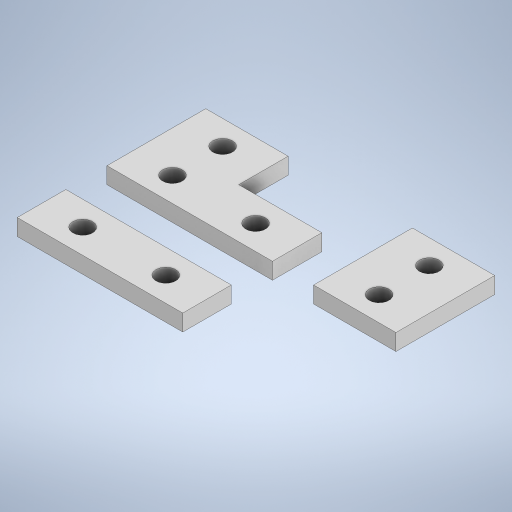
# Autodesk Inventor part: LatchBankGussetSet
Saved by Autodesk Inventor 2024 (Build 280153000, 153)
## iProperties
Created: 2023-11-04
Part Number: LatchBankGussetSet
Material: Generic
Document SubType Name: Modeling
Designer: gcter
Density: 1 g/cm^3
Appearance: Default
Author: gcter
Autodesk Inventor part; units mm, degrees
ref_plane "YZ Plane" through (0, 0, 0) normal (1, 0, 0) x (0, 1, 0)
ref_plane "XZ Plane" through (0, 0, 0) normal (0, 1, 0) x (-1, 0, 0)
ref_plane "XY Plane" through (0, 0, 0) normal (0, 0, 1) x (1, 0, 0)
sketch "Sketch1" plane through (0, 0, 0) normal (0, 1, 0) x (-1, 0, 0)
  line L0 (0, 0) -> (-25.527, 0)
  line L1 (-25.527, 0) -> (-25.527, -7.493)
  line L2 (-25.527, -7.493) -> (0, -7.493)
  line L3 (0, -7.493) -> (0, 0)
  circle A0 centre (-6.35, -3.7465) radius 1.524
  circle A1 centre (-19.177, -3.7465) radius 1.524
  line L4 (-12.7, -21.463) -> (-25.527, -21.463)
  line L5 (-25.527, -21.463) -> (-25.527, -13.843)
  line L6 (-25.527, -13.843) -> (0, -13.843)
  line L7 (0, -13.843) -> (0, -21.463)
  line L8 (0, -29.083) -> (-12.7, -29.083)
  line L9 (-12.7, -29.083) -> (-12.7, -21.463)
  line L10 (0, -21.463) -> (0, -29.083)
  circle A2 centre (-6.35, -17.5895) radius 1.524
  circle A3 centre (-19.177, -17.5895) radius 1.524
  circle A4 centre (-6.35, -25.3365) radius 1.524
  line L11 (-31.877, -13.843) -> (-44.577, -13.843)
  line L12 (-44.577, -13.843) -> (-44.577, -29.083)
  line L13 (-44.577, -29.083) -> (-31.877, -29.083)
  line L14 (-31.877, -29.083) -> (-31.877, -13.843)
  circle A5 centre (-38.227, -17.5895) radius 1.524
  circle A6 centre (-38.227, -25.3365) radius 1.524
  point P0 (-25.527, -17.653)
  dimension "d1" = 7.493
  dimension "d2" = 25.527
  dimension "d3" = 3.048
  dimension "d4" = 3.7465
  dimension "d5" = 6.35
  dimension "d6" = 6.35
  dimension "d8" = 3.048
  dimension "d9" = 6.35
  dimension "d10" = 7.62
  dimension "d11" = 7.62
  dimension "d12" = 12.7
  dimension "d13" = 3.048
  dimension "d14" = 6.35
  dimension "d15" = 3.7465
  dimension "d16" = 3.048
  dimension "d17" = 6.35
  dimension "d18" = 3.048
  dimension "d19" = 3.7465
  dimension "d20" = 12.7
  dimension "d21" = 6.35
  dimension "d22" = 3.048
  dimension "d23" = 6.35
  dimension "d24" = 3.7465
  dimension "d25" = 3.048
  dimension "d26" = 3.7465
  constraints: 30 end point, 7 centre point, 7 parallel, 5 collinear, 4 horizontal, 4 perpendicular, 2 horizontal alignment, 2 vertical alignment, 1 midpoint
  measures "d1" distance between parallel lines of L0 L2
  measures "d2" distance between parallel lines of L1 L3
  measures "d3" diameter of A0
  measures "d4" distance from line of L0 A0.centre
  measures "d5" distance from line of L3 A0.centre
  measures "d6" distance from line of A1.centre L1
  measures "d8" diameter of A1
  measures "d9" distance between parallel lines of L2 L6
  measures "d10" distance between parallel lines of L6 L4
  measures "d11" distance between parallel lines of L4 L8
  measures "d12" distance between parallel lines of L9 L10
  measures "d13" diameter of A2
  measures "d14" distance from line of L7 A2.centre
  measures "d15" distance from line of L6 A2.centre
  measures "d16" diameter of A3
  measures "d17" horizontal distance of point (-25.527, -17.653) A3.centre
  measures "d18" diameter of A4
  measures "d19" distance from line of L8 A4.centre
  measures "d20" distance between parallel lines of L12 L14
  measures "d21" distance between parallel lines of L5 L14
  measures "d22" diameter of A5
  measures "d23" distance from line of L14 A5.centre
  measures "d24" distance from line of L11 A5.centre
  measures "d25" diameter of A6
  measures "d26" distance from line of L13 A6.centre
extrude "Extrusion1" add sketch "Sketch1" along normal blind 2.54
body "Solid1"
